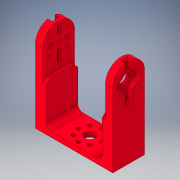
# Autodesk Inventor part: EDMO1-1_Arm
Saved by Autodesk Inventor 2019 (Build 230136000, 136)
## iProperties
Created: 2016-10-25
Part Number: EDMO1-1_Arm
Material: PLA
Document SubType Name: Modeling
Designer: Lucas
Density: 1.29985 g/cm^3
Appearance: Generic(1)
Mass: 51.3187 g
Surface Area: 168.678 cm^2
Volume: 39.4805 cm^3
Author: Lucas
Autodesk Inventor part; units mm, degrees
ref_plane "YZ Plane" through (0, 0, 0) normal (1, 0, 0) x (0, 1, 0)
sketch "Sketch1" plane through (0, 0, 0) normal (0, 0, 1) x (1, 0, 0)
  line L0 (0, 0) -> (53, 0)
  line L1 (53, 0) -> (53, 79)
  line L2 (53, 79) -> (63, 79)
  line L3 (63, 79) -> (63, -5)
  line L4 (63, -5) -> (-10, -5)
  line L5 (-10, -5) -> (-10, 79)
  line L6 (-10, 79) -> (0, 79)
  line L7 (0, 79) -> (0, 0)
  dimension "d0" = 53
  dimension "d1" = 79
  dimension "d2" = 10
  dimension "d13" = 5
  dimension "d64" = 10
  constraints: 16 end point, 5 perpendicular, 2 point on line, 1 horizontal, 1 vertical
  measures "d0" distance of L0.start L0.end
  measures "d1" distance of L0.end L1.end
  measures "d2" distance of L1.end L2.end
  measures "d13" distance between parallel lines of L4 L0
  measures "d64" distance of L5.end L6.end
extrude "Arm_Body" add sketch "Sketch1" along normal blind 30
sketch "Sketch2" plane through (63, -5, 0) normal (1, 0, 0) x (0, 0, -1)
  circle A0 centre (-15, 67) radius 1.55
  line L0 (-15, 55.5625) -> (-15, -8.8186) construction
  line L1 (-30, 0) -> (-30, 84) projected
  line L2 (0, 84) -> (0, 0) projected
  line L3 (0, 84) -> (-30, 84) projected
  point P0 (0, 5)
  dimension "d7" = 3.1
  dimension "d8" = 30
  dimension "d9" = 15
  dimension "d10" = 17
  constraints: 2 end point, 1 centre point, 1 point on line, 1 vertical
  measures "d7" diameter of A0
  measures "d8" distance between parallel lines of L1 L2
  measures "d9" distance between parallel lines of L0 L2
  measures "d10" distance from line of A0.centre L3
extrude "Shaft_Hole" cut sketch "Sketch2" against normal up to surface (73 mm away)
sketch "Sketch3" plane through (63, -5, 0) normal (1, 0, 0) x (0, 0, -1)
  circle A0 centre (-15, 67) radius 4.25
  circle A1 centre (-15, 67) radius 1.55 projected
  point P0 (0, 5)
  dimension "d14" = 8.5
  constraints: 1 centre point, 1 concentric
  measures "d14" diameter of A0
extrude "Servo_Horn_Hole" cut sketch "Sketch3" against normal up to surface (10 mm away)
sketch "Sketch4" plane through (-10, -5, 0) normal (-1, 0, 0) x (0, 0, 1)
  circle A0 centre (15, 67) radius 5
  circle A1 centre (15, 67) radius 1.55 projected
  point P0 (0, 5)
  dimension "d18" = 10
  constraints: 1 centre point, 1 concentric
  measures "d18" diameter of A0
extrude "Extrusion4" cut sketch "Sketch4" against normal blind 4.5
sketch "Sketch6" plane through (0, 0, 0) normal (0, 1, 0) x (1, 0, 0)
  circle A0 centre (26.5, -15) radius 11 construction
  line L0 (0, -15) -> (46.0375, -15)
  line L1 (53, -30) -> (0, -30) projected
  line L2 (0, 0) -> (53, 0) projected
  line L3 (0, 0) -> (0, -30) projected
  line L4 (53, 0) -> (53, -30) projected
  circle A1 centre (15.5, -15) radius 1.8
  circle A2 centre (37.5, -15) radius 1.8
  line L5 (12.9716, -1.4716) -> (40.7642, -29.2642) construction
  line L6 (12.808, -28.692) -> (38.7154, -2.7846) construction
  line L7 (26.5, 2.3185) -> (26.5, -31.0285) construction
  circle A3 centre (18.7218, -7.2218) radius 1.8
  circle A4 centre (26.5, -4) radius 1.8
  circle A5 centre (34.2782, -7.2218) radius 1.8
  circle A6 centre (26.5, -26) radius 1.8
  circle A7 centre (18.7218, -22.7782) radius 1.8
  circle A8 centre (34.2782, -22.7782) radius 1.8
  dimension "d21" = 22
  dimension "d22" = 30
  dimension "d23" = 15
  dimension "d24" = 26.5
  dimension "d25" = 53
  dimension "d26" = 3.6
  dimension "d27" = 3.6
  dimension "d28" = 45
  dimension "d29" = 45
  dimension "d30" = 90
  dimension "d31" = 3.6
  dimension "d32" = 3.6
  dimension "d33" = 3.6
  dimension "d34" = 3.6
  dimension "d35" = 3.6
  dimension "d36" = 3.6
  constraints: 12 point on line, 8 centre point, 8 end point, 1 horizontal, 10 other
  measures "d22" distance between parallel lines of L1 L2
  measures "d23" distance between parallel lines of L2 L0
  measures "d24" distance from line of point (26.5, -15) L3
  measures "d25" distance between parallel lines of L4 L3
  measures "d26" diameter of A1
  measures "d27" diameter of A2
  measures "d28" angle of L5 L0
  measures "d29" angle of L0 L6
  measures "d30" angle of L0 L7
  measures "d31" diameter of A3
  measures "d32" diameter of A4
  measures "d33" diameter of A5
  measures "d34" diameter of A6
  measures "d35" diameter of A7
  measures "d36" diameter of A8
extrude "Connector_Holes_Front" cut sketch "Sketch6" against normal up to surface (5 mm away) contours A1 L0 | L0 A1 | A2 L0 | L0 A2 | A3 | A4 | A5 | A6 | A7 | A8
fillet "Fillet9" radius 15 4 edges at (-5, 79, 0) (-5, 79, 30) (58, 79, 0) (58, 79, 30)
sketch "Sketch11" plane through (-10, -5, 0) normal (-1, 0, 0) x (0, 0, 1)
  circle A0 centre (15, 67) radius 11 construction
  circle A1 centre (15, 67) radius 1.55 projected
  line L0 (1.3636, 53.3636) -> (45.6005, 97.6005) construction
  line L1 (1.3398, 80.6602) -> (31.9798, 50.0202) construction
  line L2 (15, 36.8128) -> (15, 93.9107)
  circle A2 centre (7.2218, 59.2218) radius 1.5
  circle A3 centre (7.2218, 74.7782) radius 1.5
  circle A4 centre (22.7782, 59.2218) radius 1.5
  circle A5 centre (22.7782, 74.7782) radius 1.5
  point P0 (0, 5)
  dimension "d98" = 22
  dimension "d99" = 45
  dimension "d100" = 45
  dimension "d101" = 3
  dimension "d102" = 3
  dimension "d103" = 3
  dimension "d104" = 3
  constraints: 7 point on line, 6 end point, 5 centre point, 4 point on circle, 1 concentric, 1 vertical
  measures "d98" diameter of A0
  measures "d99" angle of L2 L0
  measures "d100" angle of L2 L1
  measures "d101" diameter of A2
  measures "d102" diameter of A3
  measures "d103" diameter of A4
  measures "d104" diameter of A5
extrude "Connector_Holes_Sides" cut sketch "Sketch11" against normal up to surface (73 mm away) contours A2 | A3 | A4 | A5
sketch "Sketch12" plane through (-10, -5, 0) normal (0, -1, 0) x (1, 0, 0)
  circle A0 centre (36.5, 15) radius 5
  line L0 (0, 0) -> (0, 30) projected
  line L1 (73, 0) -> (73, 30) projected
  line L2 (73, 0) -> (0, 0) projected
  line L3 (0, 30) -> (73, 30) projected
  point P0 (10, 0)
  dimension "d113" = 10
  dimension "d114" = 73
  dimension "d115" = 36.5
  dimension "d116" = 30
  dimension "d117" = 15
  constraints: 1 centre point
  measures "d113" diameter of A0
  measures "d114" distance between parallel lines of L0 L1
  measures "d115" distance from line of A0.centre L1
  measures "d116" distance between parallel lines of L2 L3
  measures "d117" distance from line of L3 A0.centre
extrude "Center_Hole_Front" cut sketch "Sketch12" against normal up to surface (5 mm away) contours A0
fillet "Fillet11" radius 5 2 edges at (53, 0, 15) (0, 0, 15)
sketch "Sketch22" plane through (0, 64, 15) normal (1, 0, 0) x (0, 0, -1)
  circle A0 centre (0, -2) radius 8 construction
  circle A1 centre (0, -2) radius 1.55 construction
  line L0 (30.1903, -6.25) -> (-23.8714, -6.25) construction
  line L1 (27.248, -6) -> (-22.2429, -6) construction
  line L2 (15, -59) -> (15, 0) projected
  line L3 (19.5, 5.147) -> (19.5, -12.6585) construction
  line L4 (16.5, 7.9766) -> (16.5, -20.9045) construction
  line L5 (6.7777, -6.25) -> (19.5, -5.9229)
  line L6 (-19.5, 14.6032) -> (-19.5, -22.9266) construction
  line L7 (0, -2) -> (-19.5, -2) construction
  line L8 (-6.7777, -6.25) -> (-19.5, -5.9229)
  line L9 (-16.5, 8.7128) -> (-16.5, -14.2966) construction
  line L10 (4.25, 17.6499) -> (4.25, -33.3605) construction
  line L11 (-4.25, 17.0542) -> (-4.25, -33.3605) construction
  line L12 (3, 17.0542) -> (3, -32.7841) construction
  line L13 (-3, 17.6499) -> (-3, -32.7841) construction
  line L14 (7.2088, -23) -> (-18.5055, -23) construction
  line L15 (7.2088, -18.5) -> (-15.3235, -18.5) construction
  line L16 (-15, -59) -> (-15, 0) projected
  line L17 (4.25, -8.7777) -> (2.4214, -23)
  line L18 (-4.25, -8.7777) -> (-2.4214, -23)
  line L19 (2.4214, -23) -> (-2.4214, -23)
  line L20 (19.5, -5.9229) -> (19.5, 23)
  line L21 (19.5, 23) -> (-19.5, 23)
  line L22 (-19.5, 23) -> (-19.5, -5.9229)
  circle A2 centre (0, -2) radius 1.55 projected
  circle A3 centre (0, -2) radius 7 construction
  arc A4 (6.7777, -6.25) -> (4.25, -8.7777) centre (6.6476, -8.6476) ccw
  arc A5 (-4.25, -8.7777) -> (-6.7777, -6.25) centre (-6.6476, -8.6476) ccw
  line L23 (15, -59) -> (-15, -59) projected
  point P0 (15, -64)
  point P1 (16.5, -6)
  point P2 (-16.5, -6)
  point P3 (3, -18.5)
  point P4 (-3, -18.5)
  dimension "d231" = 16
  dimension "d233" = 4.25
  dimension "d234" = 4
  dimension "d235" = 19.5
  dimension "d236" = 16.5
  dimension "d237" = 19.5
  dimension "d238" = 16.5
  dimension "d239" = 8.5
  dimension "d240" = 4.25
  dimension "d241" = 6
  dimension "d242" = 3
  dimension "d243" = 21
  dimension "d244" = 16.5
  dimension "d246" = 25
  dimension "d249" = 14
  constraints: 42 end point, 24 point on line, 8 point on circle, 5 vertical, 4 centre point, 4 parallel, 4 perpendicular, 2 collinear, 2 horizontal, 2 tangent, 1 coincident, 1 concentric
  measures "d231" diameter of A0
  measures "d233" distance from line of L0 A0.centre
  measures "d234" distance from line of L1 A0.centre
  measures "d235" distance from line of L3 A0.centre
  measures "d236" distance from line of L4 A0.centre
  measures "d237" distance from line of A0.centre L6
  measures "d238" distance from line of A0.centre L9
  measures "d239" distance between parallel lines of L10 L11
  measures "d240" distance from line of L10 A0.centre
  measures "d241" distance between parallel lines of L12 L13
  measures "d242" distance from line of L12 A0.centre
  measures "d243" distance from line of L14 A0.centre
  measures "d244" distance from line of L15 L7.start
  measures "d246" distance from line of A0.centre L21
  measures "d249" diameter of A3
extrude "Indent_Sides" cut sketch "Sketch22" against normal blind 3 contours L5 A4 L17 L19 L18 A5 L8 L22 L21 L20 | A2
ref_plane "Work Plane7" through (26.5, 64, 15) normal (1, 0, 0) x (0, 0, -1)
mirror "Mirror13" about plane through (26.5, 64, 15) normal (1, 0, 0) of "Indent_Sides"
fillet "Fillet16" radius 2.6 2 edges at (-1.5, 41, 17.4214) (-1.5, 41, 12.5786)
mirror "Mirror14" about plane through (26.5, 64, 15) normal (1, 0, 0) of "Fillet16"
sketch "Sketch26" plane through (-3, 64, 15) normal (1, 0, 0) x (0, 0, -1)
  line L0 (0, -19) -> (0, -9) construction
  line L1 (1.5, -19) -> (1.5, -9)
  line L2 (-1.5, -9) -> (-1.5, -19)
  arc A0 (-1.5, -19) -> (1.5, -19) centre (0, -19) ccw
  arc A1 (1.5, -9) -> (-1.5, -9) centre (0, -9) ccw
  circle A2 centre (0, -2) radius 1.55 construction
  line L3 (0, 21.884) -> (0, -32.2389) construction
  line L4 (0, 5) -> (0, 11) construction
  line L5 (1.5, 5) -> (1.5, 11)
  line L6 (-1.5, 11) -> (-1.5, 5)
  arc A3 (-1.5, 5) -> (1.5, 5) centre (0, 5) ccw
  arc A4 (1.5, 11) -> (-1.5, 11) centre (0, 11) ccw
  line L7 (15.7853, -2) -> (-33.0996, -2) construction
  circle A5 centre (7.5, -2) radius 2
  circle A6 centre (-7.5, -2) radius 2
  point P0 (15, -64)
  point P1 (0, -14)
  point P2 (0, 8)
  dimension "d259" = 3
  dimension "d260" = 10
  dimension "d261" = 7
  dimension "d262" = 3
  dimension "d263" = 6
  dimension "d264" = 7
  dimension "d284" = 4
  dimension "d285" = 4
  dimension "d286" = 7.5
  dimension "d287" = 7.5
  constraints: 20 end point, 8 point on circle, 8 tangent, 7 point on line, 6 centre point, 2 midpoint, 2 parallel, 2 vertical, 1 horizontal
  measures "d259" diameter of A1
  measures "d260" distance of L0.end L0.start
  measures "d261" distance of A2.centre L0.end
  measures "d262" diameter of A4
  measures "d263" distance of L4.end L4.start
  measures "d264" distance of L4.start A2.centre
  measures "d284" diameter of A5
  measures "d285" diameter of A6
  measures "d286" distance of A5.centre A2.centre
  measures "d287" distance of A6.centre A2.centre
extrude "Opening_ServoHorn_Screws" cut sketch "Sketch26" against normal up to surface (7 mm away)
mirror "Mirror16" about plane through (26.5, 64, 15) normal (1, 0, 0) of "Opening_ServoHorn_Screws"
sketch "Sketch27" plane through (-10, 64, 15) normal (-1, 0, 0) x (0, 0, 1)
  line L0 (0, -19) -> (0, 26) construction
  line L1 (3.5, -19) -> (3.5, 26)
  line L2 (-3.5, 26) -> (-3.5, -19)
  arc A0 (-3.5, -19) -> (3.5, -19) centre (0, -19) ccw
  arc A1 (3.5, 26) -> (-3.5, 26) centre (0, 26) ccw
  circle A2 centre (0, -2) radius 1.55 projected
  arc A3 (-1.5, -19) -> (1.5, -19) centre (0, -19) ccw projected
  point P0 (-15, -64)
  point P1 (0, 3.5)
  dimension "d273" = 7
  dimension "d274" = 45
  dimension "d276" = 0
  constraints: 8 end point, 4 point on circle, 4 tangent, 2 centre point, 1 midpoint, 1 parallel, 1 point on line, 1 vertical
  measures "d273" diameter of A1
  measures "d274" distance of L0.end L0.start
  measures "d276" distance of A3.centre L0.start
extrude "Pocket_ServoHorn_Screws" cut sketch "Sketch27" against normal blind 4.5
sketch "Sketch31" plane through (-10, 0, 0) normal (-1, 0, 0) x (0, 0, 1)
  circle A0 centre (7.5, 62) radius 2 construction
  circle A1 centre (7.5, 62) radius 4
  circle A2 centre (22.5, 62) radius 4
  circle A3 centre (22.5, 62) radius 2 construction
  point P0 (0, 0)
  dimension "d290" = 8
  dimension "d291" = 8
  constraints: 2 centre point, 1 coincident, 1 concentric
  measures "d290" diameter of A1
  measures "d291" diameter of A2
extrude "Extrusion27" cut sketch "Sketch31" against normal blind 4.5
mirror "Mirror19" about plane through (26.5, 64, 15) normal (1, 0, 0) of "Extrusion4"
mirror "Mirror20" about plane through (26.5, 64, 15) normal (1, 0, 0) of "Pocket_ServoHorn_Screws", "Extrusion27"
sketch "Sketch32" plane through (0, 5, 30) normal (1, 0, 0) x (0, 0, -1)
  line L0 (30, 74) -> (0, 74)
  line L1 (0, 74) -> (0, 34)
  line L2 (0, 34) -> (30, 34)
  line L3 (30, 34) -> (30, 74)
  line L4 (24.1782, 45.2218) -> (18.6071, 45.2218) projected
  line L5 (30, 52.9614) -> (30, 0) projected
  line L6 (0, 0) -> (0, 52.9614) projected
  arc A0 (30, 59) -> (0, 59) centre (15, 59) ccw projected
  point P0 (30, -5)
  point P1 (14.8657, 36)
  dimension "d307" = 2
  constraints: 8 end point, 2 collinear, 2 parallel, 1 horizontal, 1 perpendicular, 1 tangent
  measures "d307" distance from line of L2 point (14.866, 36)
extrude "Indentation_Sides_Inside_right" cut sketch "Sketch32" against normal blind 3
ref_plane "Work Plane8" through (26.5, -5, 0) normal (-1, 0, 0) x (0, 0, 1)
sketch "Sketch33" plane through (53, 5, 0) normal (-1, 0, 0) x (0, 0, 1)
  line L0 (30, 74) -> (0, 74)
  line L1 (0, 74) -> (0, 34)
  line L2 (0, 34) -> (30, 34)
  line L3 (30, 34) -> (30, 74)
  arc A0 (30, 59) -> (0, 59) centre (15, 59) ccw projected
  line L4 (0, 0) -> (0, 52.9614) projected
  line L5 (30, 52.9614) -> (30, 0) projected
  line L6 (11.3929, 45.2218) -> (5.8218, 45.2218) projected
  point P0 (0, -5)
  point P1 (15.1343, 36)
  dimension "d308" = 2
  constraints: 8 end point, 2 collinear, 2 parallel, 1 horizontal, 1 perpendicular, 1 tangent
  measures "d308" distance from line of L2 point (15.134, 36)
extrude "Indentation_Sides_Inside_left" cut sketch "Sketch33" against normal blind 3
chamfer "Chamfer4" distance 4 angle 45 4 edges at (-1.5, 39, 30) (-1.5, 39, 0) (54.5, 39, 30) (54.5, 39, 0)
sketch "Sketch34" plane through (63, -5, 30) normal (1, 0, 0) x (0, 0, -1)
  arc A0 (10.65, 69.4653) -> (10.65, 64.5347) centre (7.5, 67) ccw projected
  line L0 (7.5, 71) -> (11.5, 75)
  line L1 (11.5, 83.586) -> (11.5, 70.5707) projected
  line L2 (7.5, 71) -> (13.1569, 71) construction
  line L3 (11.5, 75) -> (18.5, 75)
  line L4 (18.5, 75) -> (22.5, 71)
  arc A1 (19.35, 64.5347) -> (19.35, 69.4653) centre (22.5, 67) ccw projected
  line L5 (18.5, 50) -> (18.5, 63.4293) projected
  line L6 (7.5, 71) -> (7.5, 67)
  line L7 (7.5, 67) -> (22.5, 67) construction
  line L8 (22.5, 67) -> (22.5, 71)
  line L9 (7.5, 63) -> (11.5, 59)
  line L10 (11.5, 59) -> (18.5, 59)
  line L11 (18.5, 59) -> (22.5, 63)
  line L12 (7.5, 63) -> (7.5, 67)
  line L13 (22.5, 67) -> (22.5, 63)
  point P0 (30, 5)
  dimension "d312" = 45
  constraints: 24 end point, 4 symmetric about line, 2 perpendicular, 2 point on circle, 2 point on line, 2 vertical, 1 equal length, 1 horizontal
  measures "d312" angle of L2 L0
extrude "Extrusion30" cut sketch "Sketch34" against normal up to surface (4.5 mm away) contours L0 L3 L4 L8 L13 L11 L10 L9 L12 L6
mirror "Mirror21" about plane through (26.5, -5, 0) normal (-1, 0, 0) of "Extrusion30"
sketch "Sketch35" plane through (-10, -5, 0) normal (0, -1, 0) x (1, 0, 0)
  line L0 (1.7396, 30.0008) -> (27.5293, 30.0008) construction
  line L1 (27.5293, 30.0008) -> (27.5293, 0.0394) construction
  line L2 (27.5293, 0.0394) -> (1.7396, 0.0394) construction
  line L3 (1.7396, 0.0394) -> (1.7396, 30.0008) construction
  line L4 (28.4581, 31.6534) -> (28.4581, 1.5619) construction
  line L5 (42.4254, 30.2009) -> (73.22, 30.2009) construction
  line L6 (73.22, 30.2009) -> (73.22, -0.3361) construction
  line L7 (73.22, -0.3361) -> (42.4254, -0.3361) construction
  line L8 (42.4254, -0.3361) -> (42.4254, 30.2009) construction
  line L9 (2.6731, 18.024) -> (2.6731, 27.024)
  line L10 (2.6731, 27.024) -> (8.7558, 27.024)
  line L11 (8.7558, 27.024) -> (8.7558, 25.3101)
  line L12 (8.7558, 25.3101) -> (4.9195, 25.3101)
  line L13 (4.9195, 25.3101) -> (4.9195, 23.7274)
  line L14 (4.9195, 23.7274) -> (8.4567, 23.7274)
  line L15 (8.4567, 23.7274) -> (8.4567, 22.0135)
  line L16 (8.4567, 22.0135) -> (4.9195, 22.0135)
  line L17 (4.9195, 22.0135) -> (4.9195, 19.738)
  line L18 (4.9195, 19.738) -> (8.7558, 19.738)
  line L19 (8.7558, 19.738) -> (8.7558, 18.024)
  line L20 (8.7558, 18.024) -> (2.6731, 18.024)
  spline S0 degree 2 poles (18.3174, 22.5167) (18.3174, 21.255) (17.2161, 19.2712) (16.3773, 18.7388) knots 0 0 0 1 2 2 2
  spline S1 degree 2 poles (16.3773, 18.7388) (15.6772, 18.2866) (14.0289, 18.024) (13.1026, 18.024) knots 0 0 0 1 2 2 2
  line L21 (13.1026, 18.024) -> (10.2874, 18.024)
  line L22 (10.2874, 18.024) -> (10.2874, 27.024)
  line L23 (10.2874, 27.024) -> (13.0734, 27.024)
  spline S2 degree 2 poles (13.0734, 27.024) (14.0216, 27.024) (15.6772, 26.7833) (16.4065, 26.3166) knots 0 0 0 1 2 2 2
  spline S3 degree 2 poles (16.4065, 26.3166) (17.289, 25.7477) (18.3174, 23.8222) (18.3174, 22.5167) knots 0 0 0 1 2 2 2
  spline S4 degree 2 poles (15.9981, 22.5313) (15.9981, 23.4211) (15.3854, 24.6901) (14.7582, 25.0475) knots 0 0 0 1 2 2 2
  spline S5 degree 2 poles (14.7582, 25.0475) (14.2987, 25.2955) (13.2922, 25.3465) (12.5921, 25.3465) knots 0 0 0 1 2 2 2
  line L24 (12.5921, 25.3465) -> (12.5483, 25.3465)
  line L25 (12.5483, 25.3465) -> (12.5483, 19.7088)
  line L26 (12.5483, 19.7088) -> (12.5921, 19.7088)
  spline S6 degree 2 poles (12.5921, 19.7088) (13.3506, 19.7088) (14.3935, 19.7598) (14.8676, 20.0589) knots 0 0 0 1 2 2 2
  spline S7 degree 2 poles (14.8676, 20.0589) (15.4219, 20.4089) (15.9981, 21.6415) (15.9981, 22.5313) knots 0 0 0 1 2 2 2
  line L27 (11.8627, 3.2058) -> (9.6164, 3.2058)
  line L28 (9.6164, 3.2058) -> (9.6164, 9.1717)
  line L29 (9.6164, 9.1717) -> (7.9827, 5.3208)
  line L30 (7.9827, 5.3208) -> (6.4365, 5.3208)
  line L31 (6.4365, 5.3208) -> (4.8028, 9.1717)
  line L32 (4.8028, 9.1717) -> (4.8028, 3.2058)
  line L33 (4.8028, 3.2058) -> (2.6731, 3.2058)
  line L34 (2.6731, 3.2058) -> (2.6731, 12.2058)
  line L35 (2.6731, 12.2058) -> (5.2768, 12.2058)
  line L36 (5.2768, 12.2058) -> (7.2752, 7.7641)
  line L37 (7.2752, 7.7641) -> (9.259, 12.2058)
  line L38 (9.259, 12.2058) -> (11.8627, 12.2058)
  line L39 (11.8627, 12.2058) -> (11.8627, 3.2058)
  spline S8 degree 2 poles (21.9203, 7.7058) (21.9203, 5.5177) (19.5864, 3.0161) (17.5589, 3.0161) knots 0 0 0 1 2 2 2
  spline S9 degree 2 poles (17.5589, 3.0161) (15.524, 3.0161) (13.2047, 5.5469) (13.2047, 7.7058) knots 0 0 0 1 2 2 2
  spline S10 degree 2 poles (13.2047, 7.7058) (13.2047, 9.8719) (15.524, 12.3954) (17.5589, 12.3954) knots 0 0 0 1 2 2 2
  spline S11 degree 2 poles (17.5589, 12.3954) (19.5864, 12.3954) (21.9203, 9.8865) (21.9203, 7.7058) knots 0 0 0 1 2 2 2
  spline S12 degree 2 poles (19.5864, 7.7058) (19.5864, 8.5153) (19.2582, 9.6458) (18.9738, 10.0032) knots 0 0 0 1 2 2 2
  spline S13 degree 2 poles (18.9738, 10.0032) (18.6893, 10.3751) (17.96, 10.696) (17.5661, 10.696) knots 0 0 0 1 2 2 2
  spline S14 degree 2 poles (17.5661, 10.696) (17.1504, 10.696) (16.4721, 10.397) (16.1585, 10.0177) knots 0 0 0 1 2 2 2
  spline S15 degree 2 poles (16.1585, 10.0177) (15.8814, 9.6677) (15.5386, 8.508) (15.5386, 7.7058) knots 0 0 0 1 2 2 2
  spline S16 degree 2 poles (15.5386, 7.7058) (15.5386, 6.8743) (15.8668, 5.7803) (16.1512, 5.4083) knots 0 0 0 1 2 2 2
  spline S17 degree 2 poles (16.1512, 5.4083) (16.4357, 5.0364) (17.1723, 4.7155) (17.5661, 4.7155) knots 0 0 0 1 2 2 2
  spline S18 degree 2 poles (17.5661, 4.7155) (17.9673, 4.7155) (18.7112, 5.0583) (18.9811, 5.4229) knots 0 0 0 1 2 2 2
  spline S19 degree 2 poles (18.9811, 5.4229) (19.2728, 5.8168) (19.5864, 6.8597) (19.5864, 7.7058) knots 0 0 0 1 2 2 2
  spline S20 degree 2 poles (62.1002, 22.9251) (62.1002, 21.6634) (60.9989, 19.6796) (60.1602, 19.1471) knots 0 0 0 1 2 2 2
  spline S21 degree 2 poles (60.1602, 19.1471) (59.46, 18.695) (57.8118, 18.4324) (56.8855, 18.4324) knots 0 0 0 1 2 2 2
  line L40 (56.8855, 18.4324) -> (54.0703, 18.4324)
  line L41 (54.0703, 18.4324) -> (54.0703, 27.4324)
  line L42 (54.0703, 27.4324) -> (56.8563, 27.4324)
  spline S22 degree 2 poles (56.8563, 27.4324) (57.8045, 27.4324) (59.46, 27.1917) (60.1894, 26.7249) knots 0 0 0 1 2 2 2
  spline S23 degree 2 poles (60.1894, 26.7249) (61.0719, 26.1561) (62.1002, 24.2306) (62.1002, 22.9251) knots 0 0 0 1 2 2 2
  spline S24 degree 2 poles (59.781, 22.9397) (59.781, 23.8295) (59.1683, 25.0985) (58.5411, 25.4559) knots 0 0 0 1 2 2 2
  spline S25 degree 2 poles (58.5411, 25.4559) (58.0816, 25.7039) (57.0751, 25.7549) (56.375, 25.7549) knots 0 0 0 1 2 2 2
  line L43 (56.375, 25.7549) -> (56.3312, 25.7549)
  line L44 (56.3312, 25.7549) -> (56.3312, 20.1172)
  line L45 (56.3312, 20.1172) -> (56.375, 20.1172)
  spline S26 degree 2 poles (56.375, 20.1172) (57.1335, 20.1172) (58.1764, 20.1682) (58.6505, 20.4672) knots 0 0 0 1 2 2 2
  spline S27 degree 2 poles (58.6505, 20.4672) (59.2048, 20.8173) (59.781, 22.0499) (59.781, 22.9397) knots 0 0 0 1 2 2 2
  line L46 (69.5796, 10.4324) -> (66.8446, 10.4324)
  line L47 (66.8446, 10.4324) -> (64.4013, 14.0864)
  line L48 (64.4013, 14.0864) -> (63.9564, 13.4737)
  line L49 (63.9564, 13.4737) -> (63.9564, 10.4324)
  line L50 (63.9564, 10.4324) -> (61.6955, 10.4324)
  line L51 (61.6955, 10.4324) -> (61.6955, 19.4324)
  line L52 (61.6955, 19.4324) -> (63.9564, 19.4324)
  line L53 (63.9564, 19.4324) -> (63.9564, 15.4138)
  line L54 (63.9564, 15.4138) -> (66.8446, 19.4324)
  line L55 (66.8446, 19.4324) -> (69.4483, 19.4324)
  line L56 (69.4483, 19.4324) -> (66.2392, 15.2533)
  line L57 (66.2392, 15.2533) -> (69.5796, 10.4324)
  line L58 (54.9491, 2.4324) -> (54.9491, 11.4324)
  line L59 (54.9491, 11.4324) -> (61.0318, 11.4324)
  line L60 (61.0318, 11.4324) -> (61.0318, 9.7185)
  line L61 (61.0318, 9.7185) -> (57.1955, 9.7185)
  line L62 (57.1955, 9.7185) -> (57.1955, 8.1358)
  line L63 (57.1955, 8.1358) -> (60.7327, 8.1358)
  line L64 (60.7327, 8.1358) -> (60.7327, 6.4219)
  line L65 (60.7327, 6.4219) -> (57.1955, 6.4219)
  line L66 (57.1955, 6.4219) -> (57.1955, 4.1463)
  line L67 (57.1955, 4.1463) -> (61.0318, 4.1463)
  line L68 (61.0318, 4.1463) -> (61.0318, 2.4324)
  line L69 (61.0318, 2.4324) -> (54.9491, 2.4324)
  point P0 (10, 0)
  constraints: 4 other
extrude "DKE_Label" cut sketch "Sketch35" against normal blind 2
equation "\"d64\" = d2"
equation "\"d9\" = 0.5 * d8"
equation "\"d23\" = 0.5 * d22"
equation "\"d24\" = 0.5 * d25"
body "Solid1"
